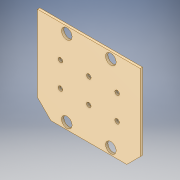
# Autodesk Inventor part: DPLX_P030_VIPE Insulation Bottom
Saved by Autodesk Inventor 2018 (Build 220112000, 112)
## iProperties
Created: 2017-12-19
Part Number: DPLX_P030_VIPE Insulation Bottom
Material: Polyethylene, High Density
Document SubType Name: Modeling
Designer: Sam
Density: 0.952 g/cm^3
Appearance: Smooth - Off-White
Mass: 5.48052 g
Surface Area: 81.4824 cm^2
Volume: 5.75685 cm^3
Author: Sam
Comments: http://www.eplastics.com/Plastic/G9-G10-FR4-glass-epoxy-sheet/G10NAT-060X12X12
Autodesk Inventor part; units mm, degrees
ref_plane "YZ Plane" through (0, 0, 0) normal (1, 0, 0) x (0, 1, 0)
ref_plane "XZ Plane" through (0, 0, 0) normal (0, 1, 0) x (-1, 0, 0)
ref_plane "XY Plane" through (0, 0, 0) normal (0, 0, 1) x (1, 0, 0)
sketch "Sketch1" plane through (0, 0, 0) normal (0, 0, 1) x (1, 0, 0)
  line L0 (-34.036, -29.7688) -> (34.036, -29.7688)
  line L1 (34.036, -29.7688) -> (34.036, 29.7688)
  line L2 (34.036, 29.7688) -> (-34.036, 29.7688)
  line L3 (-34.036, 29.7688) -> (-34.036, -29.7688)
  line L4 (-34.036, -29.7688) -> (34.036, 29.7688) construction
  line L5 (34.036, -29.7688) -> (-34.036, 29.7688) construction
  point P0 (0, 0)
  dimension "d0" = 68.072
  dimension "d1" = 59.5376
  constraints: 12 end point, 2 midpoint, 2 parallel, 1 horizontal, 1 perpendicular
  measures "d0" distance of L2.end L1.end
  measures "d1" distance of L1.end L0.end
extrude "Extrusion1" add sketch "Sketch1" along normal blind 1.524
sketch "Sketch2" plane through (0, 0, 1.524) normal (0, 0, 1) x (1, 0, 0)
  line L0 (34.036, 29.7688) -> (-34.036, 29.7688) projected
  line L1 (-34.036, -29.7688) -> (34.036, -29.7688) projected
  line L2 (-34.036, 29.7688) -> (-34.036, -29.7688) projected
  line L3 (34.036, -29.7688) -> (34.036, 29.7688) projected
  point P0 (0, 0)
  point P1 (-18.796, 8.1788)
  point P2 (-18.796, -8.1788)
  point P3 (0, 8.1788)
  point P4 (0, -8.1788)
  point P5 (18.796, 8.1788)
  point P6 (18.796, -8.1788)
  dimension "d4" = 21.59
  dimension "d5" = 21.59
  dimension "d6" = 15.24
  dimension "d7" = 15.24
  dimension "d8" = 37.592
  dimension "d9" = 18.796
  constraints: 4 horizontal alignment, 3 vertical alignment
  measures "d4" distance from line of L0 point (-18.796, 8.179)
  measures "d5" distance from line of point (-18.796, -8.179) L1
  measures "d6" distance from line of L2 point (-18.796, 8.179)
  measures "d7" distance from line of L3 point (18.796, 8.179)
  measures "d8" distance of point (18.796, 8.179) point (-18.796, 8.179)
  measures "d9" distance of point (0, 8.179) point (-18.796, 8.179)
hole "Hole1" at (-18.796, 8.1788, 1.524) at (-18.796, -8.1788, 1.524) at (0, 8.1788, 1.524) at (0, -8.1788, 1.524) at (18.796, 8.1788, 1.524) at (18.796, -8.1788, 1.524) direction (0, 0, -1) diameter 3 depth 25.4 tip angle 118
chamfer "Chamfer1" distance 8.89 angle 45 2 edges at (-34.036, -29.7688, 0.762) (34.036, -29.7688, 0.762)
sketch "Sketch4" plane through (0, 0, 1.524) normal (0, 0, 1) x (1, 0, 0)
  circle A0 centre (-14.605, 25.3976) radius 3.1496
  circle A1 centre (14.605, 25.3976) radius 3.1496
  circle A2 centre (-14.605, -25.4024) radius 3.1496
  circle A3 centre (14.605, -25.4024) radius 3.1496
  point P0 (0, 0)
  constraints: 4 centre point, 8 other
hole "Hole3" at (-14.605, 25.3976, 1.524) at (14.605, 25.3976, 1.524) at (14.605, -25.4024, 1.524) at (-14.605, -25.4024, 1.524) direction (0, 0, -1) diameter 7 end through all
equation "\"d5\" = d4"
equation "\"d7\" = d6"
equation "\"d9\" = 0.5 * d8"
body "Solid1"
